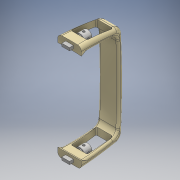
# Autodesk Inventor part: ET14
Saved by Autodesk Inventor 2016 (Build 200138000, 138)
## iProperties
Created: 2016-03-24
Part Number: ET14
Material: Genérico
Document SubType Name: Modeling
Designer: Usuario1
Density: 1 g/cm^3
Appearance: Valor por defecto
Author: Usuario1
Autodesk Inventor part; units mm, degrees
ref_plane "XZ Plane" through (0, 0, 0) normal (0, 1, 0) x (-1, 0, 0)
sketch "Boceto1" plane through (0, 0, 0) normal (1, 0, 0) x (0, 1, 0)
  line L0 (0.1061, -0.3548) -> (0, -0.4054)
  line L1 (0.1061, -5.1639) -> (0, -5.1133)
  arc A0 (1.9852, -4.7198) -> (1.9852, -0.7989) centre (-36.6887, -2.7593) ccw
  arc A1 (1.9852, -0.7989) -> (1.6867, -0.4704) centre (1.6356, -0.8166) ccw
  arc A2 (1.6867, -5.0483) -> (1.9852, -4.7198) centre (1.6356, -4.7021) ccw
  arc A3 (2.2578, -4.988) -> (2.2584, -0.5418) centre (-36.4016, -2.7593) ccw
  arc A4 (1.9192, -5.3604) -> (2.2578, -4.988) centre (1.8584, -4.965) ccw
  arc A5 (1.9266, -0.1705) -> (0, 0) centre (-0.0831, -11.9101) ccw
  arc A6 (2.2584, -0.5418) -> (1.9266, -0.1705) centre (1.8591, -0.5647) ccw
  arc A7 (0, -5.517) -> (1.9192, -5.3604) centre (-0.1413, 8.0467) ccw
  arc A8 (1.6867, -0.4704) -> (0.1061, -0.3548) centre (0.1102, -11.1677) ccw
  arc A9 (0.1061, -5.1639) -> (1.6867, -5.0483) centre (0.1102, 5.649) ccw
  line L2 (2.2545, -0.5813) -> (1.9365, -0.6471)
  line L3 (2.0303, -2.2074) -> (2.3188, -2.2074)
  arc A10 (2.3688, -2.1582) -> (2.3144, -0.626) centre (-13.0921, -1.9397) ccw
  arc A11 (2.3188, -2.2074) -> (2.3688, -2.1582) centre (2.3188, -2.1574) ccw
  arc A12 (2.3144, -0.626) -> (2.2545, -0.5813) centre (2.2646, -0.6302) ccw
  arc A13 (1.9803, -2.1581) -> (1.8969, -0.7011) centre (-14.8625, -2.3912) ccw
  arc A14 (1.9365, -0.6471) -> (1.8969, -0.7011) centre (1.9466, -0.6961) ccw
  arc A15 (1.9803, -2.1581) -> (2.0303, -2.2074) centre (2.0303, -2.1574) ccw
  line L4 (2.2545, -4.9486) -> (1.9365, -4.8828)
  line L5 (2.0303, -3.3224) -> (2.3188, -3.3224)
  arc A16 (2.3144, -4.9039) -> (2.3688, -3.3717) centre (-13.0921, -3.5902) ccw
  arc A17 (2.3688, -3.3717) -> (2.3188, -3.3224) centre (2.3188, -3.3724) ccw
  arc A18 (2.2545, -4.9486) -> (2.3144, -4.9039) centre (2.2646, -4.8997) ccw
  arc A19 (1.8969, -4.8288) -> (1.9803, -3.3717) centre (-14.8625, -3.1386) ccw
  arc A20 (1.8969, -4.8288) -> (1.9365, -4.8828) centre (1.9466, -4.8338) ccw
  arc A21 (2.0303, -3.3224) -> (1.9803, -3.3717) centre (2.0303, -3.3724) ccw
  line L6 (0, 0) -> (0, -0.4054)
  line L7 (0, -5.1133) -> (0, -5.517)
  point P0 (0, 0)
  constraints: 44 point on circle, 22 centre point, 16 end point
extrude "Extrusión1" add sketch "Boceto1" along normal blind 1.225 contours L0 L6 A5 A6 A3 A12 L2 A1 A8 | L2 A12 A3 L3 A0 A1 | L3 A3 L5 A0 | L5 A3 A18 L4 A2 A0 | L4 A18 A3 A4 A7 L7 L1 A9 A2
sketch "Boceto2" plane through (0, 0, 0) normal (0, 0, 1) x (1, 0, 0)
  line L0 (0.1828, 2.6328) -> (1.0419, 2.6328)
  arc A0 (0.1828, 2.6328) -> (0.1129, 2.5658) centre (0.1828, 2.5628) ccw
  line L1 (0, 0) -> (0.1129, 2.5658)
  line L2 (0.1888, 0.5681) -> (0.1888, 1.7493)
  arc A1 (0.2588, 1.8193) -> (0.1888, 1.7493) centre (0.2588, 1.7493) ccw
  line L3 (0.375, 0.9311) -> (0.8453, 0.9311)
  line L4 (0.8453, 0.9311) -> (0.8453, 0.5377)
  line L5 (0.375, 0.9311) -> (0.375, 0.5377)
  line L6 (0.5677, 2.7377) -> (0.2652, 2.7265)
  line L7 (0.005, 2.4396) -> (0.0114, 1.094)
  arc A2 (0.2652, 2.7265) -> (0.005, 2.4396) centre (0.2523, 2.4767) ccw
  line L8 (0.0114, 1.094) -> (0.0481, 1.0924)
  line L9 (0.5677, 2.7377) -> (0.5677, 2.6328)
  line L10 (0.2588, 0.4981) -> (0.9659, 0.4981)
  arc A3 (0.1888, 0.5681) -> (0.2588, 0.4981) centre (0.2588, 0.5681) ccw
  line L11 (0.375, 0.5377) -> (0.8453, 0.5377)
  line L12 (0.4223, 0.4981) -> (0.4223, 0.5377)
  line L13 (0.8035, 0.4981) -> (0.8035, 0.5377)
  arc A4 (1.2246, -0.0019) -> (0, 0) centre (0.5939, -11.8963) ccw
  line L14 (1.0359, 0.5681) -> (1.0359, 1.7493)
  arc A5 (1.0359, 1.7493) -> (0.9659, 1.8193) centre (0.9659, 1.7493) ccw
  line L15 (0.657, 2.7377) -> (0.9595, 2.7265)
  line L16 (1.2197, 2.4396) -> (1.2133, 1.094)
  arc A6 (1.2197, 2.4396) -> (0.9595, 2.7265) centre (0.9723, 2.4767) ccw
  line L17 (1.2133, 1.094) -> (1.1766, 1.0924)
  line L18 (0.657, 2.7377) -> (0.657, 2.6328)
  arc A7 (0.9659, 0.4981) -> (1.0359, 0.5681) centre (0.9659, 0.5681) ccw
  line L19 (0.2588, 1.8193) -> (0.9659, 1.8193)
  line L20 (0.4223, 0.4981) -> (0.8035, 0.4981)
  arc A8 (1.1118, 2.5658) -> (1.0419, 2.6328) centre (1.0419, 2.5628) ccw
  line L21 (1.2247, 0) -> (1.1118, 2.5658)
  line L22 (-0.4907, 3.227) -> (1.5675, 3.227)
  line L23 (1.5675, 3.227) -> (1.5675, -0.4444)
  line L24 (1.5675, -0.4444) -> (-0.4907, -0.4444)
  line L25 (-0.4907, -0.4444) -> (-0.4907, 3.227)
  constraints: 52 end point, 18 point on circle, 9 centre point, 8 point on line, 2 parallel, 1 horizontal, 1 perpendicular
extrude "Extrusión2" cut sketch "Boceto2" against normal blind 12.25 contours L2 A1 L19 A5 L14 A7 L10 L13 L11 L4 L3 L5 L12 A3 | L12 L11 L13 L10 | L11 L5 L3 L4
sketch "Boceto3" plane through (0, 0, 0) normal (0, 0, 1) x (1, 0, 0)
  line L0 (0.1829, 2.6346) -> (1.042, 2.6346)
  arc A0 (0.1829, 2.6346) -> (0.113, 2.5677) centre (0.1829, 2.5646) ccw
  line L1 (0.0001, 0.0019) -> (0.113, 2.5677)
  line L2 (0.1888, 0.5681) -> (0.1888, 1.7493)
  arc A1 (0.2588, 1.8193) -> (0.1888, 1.7493) centre (0.2588, 1.7493) ccw
  line L3 (0.375, 0.9311) -> (0.8453, 0.9311)
  line L4 (0.8453, 0.9311) -> (0.8453, 0.5377)
  line L5 (0.375, 0.9311) -> (0.375, 0.5377)
  line L6 (0.5678, 2.7396) -> (0.2653, 2.7284)
  line L7 (0.0051, 2.4415) -> (0.0115, 1.0959)
  arc A2 (0.2653, 2.7284) -> (0.0051, 2.4415) centre (0.2524, 2.4786) ccw
  line L8 (0.0115, 1.0959) -> (0.0482, 1.0943)
  line L9 (0.5678, 2.7396) -> (0.5678, 2.6346)
  line L10 (0.2588, 0.4981) -> (0.9659, 0.4981)
  arc A3 (0.1888, 0.5681) -> (0.2588, 0.4981) centre (0.2588, 0.5681) ccw
  line L11 (0.375, 0.5377) -> (0.8453, 0.5377)
  line L12 (0.4223, 0.4981) -> (0.4223, 0.5377)
  line L13 (0.8035, 0.4981) -> (0.8035, 0.5377)
  arc A4 (1.225, 0) -> (0.0001, 0.0019) centre (0.5945, -11.8944) ccw
  line L14 (1.0359, 0.5681) -> (1.0359, 1.7493)
  arc A5 (1.0359, 1.7493) -> (0.9659, 1.8193) centre (0.9659, 1.7493) ccw
  line L15 (0.657, 2.7395) -> (0.9595, 2.7284)
  line L16 (1.2197, 2.4396) -> (1.2136, 1.094)
  arc A6 (1.2197, 2.4396) -> (0.9595, 2.7284) centre (0.9727, 2.4786) ccw
  line L17 (1.2136, 1.094) -> (1.1768, 1.0924)
  line L18 (0.657, 2.7395) -> (0.657, 2.6346)
  arc A7 (0.9659, 0.4981) -> (1.0359, 0.5681) centre (0.9659, 0.5681) ccw
  line L19 (0.2588, 1.8193) -> (0.9659, 1.8193)
  line L20 (0.4223, 0.4981) -> (0.8035, 0.4981)
  arc A8 (1.1118, 2.5658) -> (1.042, 2.6346) centre (1.0418, 2.5646) ccw
  line L21 (1.225, 0) -> (1.1118, 2.5658)
  line L22 (0, 1.9192) -> (0, 0) projected
  line L23 (0.113, 2.5677) -> (0, 0)
  line L24 (1.1118, 2.5658) -> (1.225, 0)
  line L25 (0, 0) -> (1.225, 0) projected
  line L26 (1.225, 0) -> (1.1118, 2.5658)
  line L27 (-0.3668, 3.0653) -> (1.5665, 3.0653)
  line L28 (1.5665, 3.0653) -> (1.5665, -0.361)
  line L29 (1.5665, -0.361) -> (-0.3668, -0.361)
  line L30 (-0.3668, -0.361) -> (-0.3668, 3.0653)
  constraints: 58 end point, 18 point on circle, 9 centre point, 8 point on line, 2 collinear, 2 parallel, 1 horizontal, 1 perpendicular
extrude "Extrusión3" cut sketch "Boceto3" against normal blind 12.25 contours A0 L1 L8 L7 A2 L6 L9 L0 | L18 L15 A6 L16 L17 L21 A8 L0 | A4 L25 | L27 L28 L29 L30
ref_plane "Plano de trabajo1" through (0, 0, -0.2) normal (0, 0, 1) x (1, 0, 0)
sketch "Boceto4" plane through (0, 0, -0.2) normal (0, 0, 1) x (1, 0, 0)
  line L0 (0.0047, 0.1061) -> (0.0742, 1.6867) projected
  line L1 (0.0742, 1.6867) -> (0.1888, 1.6867) projected
  line L2 (0.1888, 1.6867) -> (0.1888, 0.5681) projected
  line L3 (0.2588, 0.4981) -> (0.9659, 0.4981) projected
  line L4 (1.0359, 0.5681) -> (1.0359, 1.6867) projected
  line L5 (1.0359, 1.6867) -> (1.1506, 1.6867) projected
  line L6 (1.1506, 1.6867) -> (1.2203, 0.1061) projected
  line L7 (0.0047, 0.1061) -> (1.2203, 0.1061) projected
  line L8 (0.375, 0.9311) -> (0.8453, 0.9311)
  line L9 (0.8453, 0.9311) -> (0.8453, 0.5377)
  line L10 (0.375, 0.9311) -> (0.375, 0.5377)
  line L11 (0.2588, 0.4981) -> (0.9659, 0.4981)
  line L12 (0.375, 0.5377) -> (0.8453, 0.5377)
  line L13 (0.4223, 0.4981) -> (0.4223, 0.5377)
  line L14 (0.8035, 0.4981) -> (0.8035, 0.5377)
  line L15 (0.4223, 0.4981) -> (0.8035, 0.4981)
  line L16 (0.2588, 0.4981) -> (0.9659, 0.4981) projected
  line L17 (0.6123, 0.4981) -> (0.6123, 1.1926)
  line L18 (0.6123, 0.9311) -> (0.8453, 0.9311)
  line L19 (0.8453, 0.9311) -> (0.8453, 0.5377)
  line L20 (0.8453, 0.5377) -> (0.6123, 0.5377)
  line L21 (0.6123, 0.5377) -> (0.6123, 0.9311)
  line L22 (0.6123, 0.5377) -> (0.8035, 0.5377)
  line L23 (0.8035, 0.5377) -> (0.8035, 0.4981)
  line L24 (0.8035, 0.4981) -> (0.6123, 0.4981)
  line L25 (0.6123, 0.4981) -> (0.6123, 0.5377)
  point P0 (0, 0)
  constraints: 34 end point, 6 point on line, 4 parallel, 2 horizontal, 2 perpendicular, 1 midpoint, 1 vertical, 2 other
revolve "Revolución1" add sketch "Boceto4" angle 360 about axis through (0.6123, 0.4981, -0.2) along (0, 1, 0) contours L17 L12 L14 L3 | L17 L8 L9 L12
sketch "Boceto5" plane through (0, 0, -0.2) normal (0, 0, 1) x (1, 0, 0)
  line L0 (0.3793, 0.9311) -> (0.8453, 0.9311) projected
  line L1 (0.3793, 0.5377) -> (0.8453, 0.5377) projected
  line L2 (0.8453, 0.9311) -> (0.8453, 0.5377) projected
  line L3 (0.3793, 0.9311) -> (0.8453, 0.9311) projected
  line L4 (0.3793, 0.5377) -> (0.8453, 0.5377) projected
  circle A0 centre (0.6123, 0.7344) radius 0.06
  point P0 (0, 0)
  constraints: 1 centre point
extrude "Extrusión4" cut sketch "Boceto5" along normal mid plane 1.25
ref_plane "Plano de trabajo2" through (0, 0, -5.32) normal (0, 0, 1) x (1, 0, 0)
sketch "Boceto6" plane through (0, 0, -5.32) normal (0, 0, 1) x (1, 0, 0)
  line L0 (0.0001, 0.0019) -> (0.0844, 1.9192) projected
  line L1 (0.0844, 1.9192) -> (1.1403, 1.9192) projected
  line L2 (1.1403, 1.9192) -> (1.225, 0) projected
  line L3 (1.0359, 0.5681) -> (1.0359, 1.7493) projected
  line L4 (0.9659, 1.8193) -> (0.2588, 1.8193) projected
  line L5 (0.1888, 1.7493) -> (0.1888, 0.5681) projected
  line L6 (0.2588, 0.4981) -> (0.9659, 0.4981) projected
  line L7 (0.1831, 2.6328) -> (1.0422, 2.6328)
  arc A0 (0.1831, 2.6328) -> (0.1132, 2.5658) centre (0.1831, 2.5628) ccw
  line L8 (0.0003, 0) -> (0.1132, 2.5658)
  line L9 (0.1891, 0.5681) -> (0.1891, 1.7493)
  arc A1 (0.2591, 1.8193) -> (0.1891, 1.7493) centre (0.2591, 1.7493) ccw
  line L10 (0.3753, 0.9311) -> (0.3753, 0.5377)
  line L11 (0.568, 2.7377) -> (0.2655, 2.7265)
  line L12 (0.0053, 2.4396) -> (0.0117, 1.094)
  arc A2 (0.2655, 2.7265) -> (0.0053, 2.4396) centre (0.2527, 2.4767) ccw
  line L13 (0.0117, 1.094) -> (0.0484, 1.0924)
  line L14 (0.568, 2.7377) -> (0.568, 2.6328)
  line L15 (0.2591, 0.4981) -> (0.9662, 0.4981)
  arc A3 (0.1891, 0.5681) -> (0.2591, 0.4981) centre (0.2591, 0.5681) ccw
  line L16 (0.4227, 0.4981) -> (0.4227, 0.5377)
  arc A4 (1.225, -0.0019) -> (0.0003, 0) centre (0.5943, -11.8963) ccw
  line L17 (1.0362, 0.5681) -> (1.0362, 1.7493)
  arc A5 (1.0362, 1.7493) -> (0.9662, 1.8193) centre (0.9662, 1.7493) ccw
  line L18 (0.6573, 2.7377) -> (0.9598, 2.7265)
  line L19 (1.22, 2.4396) -> (1.2136, 1.094)
  arc A6 (1.22, 2.4396) -> (0.9598, 2.7265) centre (0.9727, 2.4767) ccw
  line L20 (1.2136, 1.094) -> (1.1769, 1.0924)
  line L21 (0.6573, 2.7377) -> (0.6573, 2.6328)
  arc A7 (0.9662, 0.4981) -> (1.0362, 0.5681) centre (0.9662, 0.5681) ccw
  line L22 (0.2591, 1.8193) -> (0.9662, 1.8193)
  line L23 (0.4227, 0.4981) -> (0.8039, 0.4981)
  arc A8 (1.1121, 2.5658) -> (1.0422, 2.6328) centre (1.0422, 2.5628) ccw
  line L24 (1.225, 0) -> (1.1121, 2.5658)
  line L25 (0.6133, 0.4981) -> (0.4227, 0.4981)
  line L26 (0.4227, 0.4981) -> (0.4227, 0.5377)
  line L27 (0.4227, 0.5377) -> (0.6133, 0.5377)
  line L28 (0.6133, 0.5377) -> (0.6133, 0.4981)
  line L29 (0.6133, 0.5377) -> (0.3753, 0.5377)
  line L30 (0.3753, 0.5377) -> (0.3753, 0.9311)
  line L31 (0.3753, 0.9311) -> (0.6133, 0.9311)
  line L32 (0.6133, 0.9311) -> (0.6133, 0.5377)
  line L33 (0.6133, 0.4981) -> (0.6133, 1.2585)
  point P0 (0, 0)
  constraints: 54 end point, 18 point on circle, 9 centre point, 6 point on line, 4 parallel, 2 horizontal, 2 perpendicular, 1 midpoint, 1 vertical, 5 other
revolve "Revolución2" add sketch "Boceto6" angle 360 about axis through (0.6133, 0.4981, -5.32) along (0, 1, 0) contours L6 L16 L27 L28 | L27 L29 L10 L31 L32
sketch "Boceto7" plane through (0, 0, -5.32) normal (0, 0, 1) x (1, 0, 0)
  spline S0 degree 8 poles (0.6723, 0.7344) (0.6723, 0.7465) (0.6695, 0.7584) (0.6641, 0.7694) (0.6564, 0.779) (0.6467, 0.7867) (0.6355, 0.7919) (0.6238, 0.7944) (0.6009, 0.7944) (0.5891, 0.7919) (0.578, 0.7867) (0.5683, 0.779) (0.5605, 0.7694) (0.5551, 0.7584) (0.5523, 0.7465) (0.5523, 0.7223) (0.5551, 0.7104) (0.5605, 0.6993) (0.5683, 0.6897) (0.578, 0.6821) (0.5891, 0.6769) (0.6009, 0.6744) (0.6238, 0.6744) (0.6355, 0.6769) (0.6467, 0.6821) (0.6564, 0.6897) (0.6641, 0.6993) (0.6695, 0.7104) (0.6723, 0.7223) (0.6723, 0.7344) knots 0 0 0 0 0 0 0 0 0 0.25 0.25 0.25 0.25 0.25 0.25 0.25 0.5 0.5 0.5 0.5 0.5 0.5 0.5 0.75 0.75 0.75 0.75 0.75 0.75 0.75 1 1 1 1 1 1 1 1 1 projected
  point P0 (0, 0)
  constraints: 1 other
extrude "Extrusión5" cut sketch "Boceto7" along normal mid plane 1.25
ref_plane "Plano de trabajo3" through (0.61, 0, 0) normal (1, 0, 0) x (0, 1, 0)
sketch "Boceto8" plane through (0.61, 0, 0) normal (1, 0, 0) x (0, 1, 0)
  line L0 (0.9311, 0.033) -> (0.9311, -0.433) projected
  line L1 (0.9311, -0.433) -> (0.5377, -0.433) projected
  line L2 (0.9311, -0.2) -> (0.6353, -0.2)
  line L3 (0.7344, -0.433) -> (0.7344, -0.2)
  line L4 (0.5377, -5.5579) -> (0.5377, -5.0821) projected
  line L5 (0.9311, -5.5579) -> (0.9311, -5.0821) projected
  line L6 (0.9311, -5.5579) -> (0.9311, -5.0821) projected
  line L7 (0.9311, -5.32) -> (0.5377, -5.32)
  line L8 (0.7344, -5.32) -> (0.9311, -5.32)
  circle A0 centre (0.7344, -0.2) radius 0.06
  circle A1 centre (0.7344, -5.32) radius 0.06
  point P0 (0, 0)
  dimension "d16" = 0.12
  dimension "d17" = 0.12
  constraints: 8 end point, 5 midpoint, 2 centre point, 2 coincident, 1 collinear, 1 horizontal, 1 perpendicular, 1 point on line, 2 other
  measures "d16" diameter of A0
  measures "d17" diameter of A1
extrude "Extrusión6" cut sketch "Boceto8" along normal mid plane 0.55 contours A0 L3 L2 | L2 A0 | L3 A0 L2 | A1 L7 | L7 A1
fillet "Empalme1" radius 0.2 12 edges at (1.1823, 0.9667, -0.0461) (1.1298, 2.1573, -0.2982) (1.1226, 2.3219, -2.7649) (1.13, 2.1544, -5.2341) (1.1825, 0.9624, -5.4728) (0.0242, 0.5487, -0.0165) (0.0665, 1.5114, -0.1069) (0.1022, 2.3219, -2.7649) (0.0948, 2.1544, -5.2341) (0.0663, 1.5075, -5.4172) (0.0242, 0.5486, -5.5002) (0.0949, 2.1573, -0.2982)
fillet "Empalme2" radius 0.1 12 edges at (1.1352, 2.0348, -2.7593) (1.1414, 1.8947, -0.5813) (1.1854, 0.8985, -0.3836) (1.1414, 1.8947, -4.9374) (1.1854, 0.8985, -5.1351) (0.0834, 1.8947, -4.9374) (0.0264, 0.6007, -5.1527) (0.0612, 1.391, -5.0877) (0.0834, 1.8947, -0.5813) (0.0612, 1.391, -0.431) (0.0264, 0.6007, -0.366) (0.0895, 2.0348, -2.7593)
sketch "Boceto9" plane through (0, 0, 0) normal (0, 1, 0) x (-1, 0, 0)
  line L0 (-1.225, -5.1133) -> (-1.225, -5.3171) projected
  ellipse E0 centre (-0.5945, 0.5555) end of major axis (11.3167, 0.5555) minor radius 5.6767 (-1.225, -5.1133) -> (-0.0001, -5.1142) ccw projected
  line L1 (-0.0001, -5.1142) -> (-0.0001, -5.3171) projected
  line L2 (-0.0001, -0.2) -> (-0.0001, -0.4045) projected
  ellipse E1 centre (-0.5945, -6.0742) end of major axis (-12.5056, -6.0742) minor radius 5.6767 (-0.0001, -0.4045) -> (-1.225, -0.4054) ccw projected
  line L3 (-1.225, -0.1999) -> (-1.225, -0.4054) projected
  circle A0 centre (-0.6123, -0.2) radius 0.1912 projected
  line L4 (-0.0001, -5.3171) -> (-1.225, -5.3171)
  line L5 (-0.6125, -5.3171) -> (-0.4125, -5.3171)
  line L6 (-0.4125, -5.3171) -> (-0.4126, -5.2421)
  line L7 (-0.4126, -5.2421) -> (-0.8126, -5.2421)
  line L8 (-0.8126, -5.2421) -> (-0.8125, -5.3921)
  line L9 (-0.8125, -5.3921) -> (-0.4125, -5.3921)
  line L10 (-0.4125, -5.3921) -> (-0.4126, -5.2421)
  line L11 (-0.4126, -0.125) -> (-0.8126, -0.125)
  line L12 (-0.8126, -0.125) -> (-0.8125, -0.275)
  line L13 (-0.8125, -0.275) -> (-0.4125, -0.275)
  line L14 (-0.4125, -0.275) -> (-0.4126, -0.125)
  point P0 (0, 0)
  point P1 (-0.6123, -0.2)
  dimension "d22" = 0.2
  dimension "d23" = 0.075
  dimension "d24" = 0.4
  dimension "d25" = 0.15
  dimension "d26" = 0.4
  dimension "d27" = 0.4
  dimension "d28" = 0.15
  dimension "d29" = 0.4
  constraints: 22 end point, 6 perpendicular, 2 point on line, 1 midpoint, 8 other
  measures "d22" distance of L5.start L5.end
  measures "d23" distance of L5.end L6.end
  measures "d24" distance of L6.end L7.end
  measures "d25" distance of L7.end L8.end
  measures "d26" distance of L8.end L9.end
  measures "d27" distance of L14.end L11.end
  measures "d28" distance of L11.end L13.start
  measures "d29" distance of L13.start L14.start
extrude "Extrusión7" add sketch "Boceto9" against normal blind 0.2 contours L8 L7 L6 L4 | L4 L10 L9 L8 | A0 L13 L11 | A0 L11 L14 L13 | A0 L13 L12 L11
